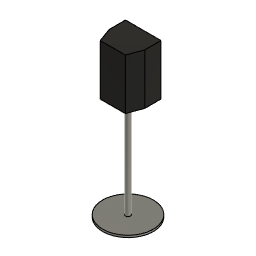
Speaker (Autodesk Fusion 360 design; units mm, degrees)
Autodesk Fusion 360 part; units mm, degrees
sketch "Schizzo1" plane through (0, 0, 0) normal (0, 0, 1) x (1, 0, 0)
  circle A0 centre (0, 0) radius 250
  dimension "d1" = 500
  constraint coincident A0.centre origin
  measures "d1" diameter of A0
extrude "Estrusione1" add sketch "Schizzo1" along normal blind 20
sketch "Schizzo2" plane through (0, 0, 20) normal (0, 0, 1) x (-1, 0, 0)
  circle A0 centre (0, 0) radius 250
  circle A1 centre (0, 0) radius 25
  dimension "d4" = 50
  constraint coincident A0.centre A1.centre
  measures "d4" diameter of A1
extrude "Estrusione2" add sketch "Schizzo2" along normal blind 1000 contours A1
sketch "Schizzo3" plane through (0, 0, 1020) normal (0, 0, 1) x (-1, 0, 0)
  circle A0 centre (0, 0) radius 25
  line L0 (-175, -150) -> (175, -150)
  line L1 (175, -150) -> (175, 150)
  line L2 (175, 150) -> (-175, 150)
  line L3 (-175, 150) -> (-175, -150)
  line L4 (-175, -150) -> (175, 150) construction
  line L5 (175, -150) -> (-175, 150) construction
  line L6 (-123.697, 150) -> (-175, 9.0461)
  line L7 (123.697, 150) -> (175, 9.0461)
  dimension "d7" = 350
  dimension "d8" = 300
  dimension "d11" = 150
  dimension "d12" = 20
  dimension "d13" = 20
  constraint horizontal L0
  constraint perpendicular L0 L1
  constraint parallel L0 L2
  constraint parallel L1 L3
  constraint coincident L4 A0.centre
  constraint coincident L5 A0.centre
  constraint coincident A0.centre origin
  constraint coincident L2 L6.start
  constraint coincident L3 L6.end
  constraint coincident L2 L7.start
  constraint coincident L1 L7.end
  constraint equal L6 L7
  measures "d7" distance of L1.end L2.end
  measures "d8" distance of L0.end L1.end
  measures "d11" distance of L6.start L6.end
  measures "d12" angle of L3 L6
  measures "d13" angle of L1 L7
extrude "Estrusione3" add sketch "Schizzo3" along normal blind 500 contours A0 | L0 L1 L2 L3 L6 L7
sketch "Schizzo4" plane through (0, 150, 0) normal (0, 1, 0) x (-1, 0, 0)
  line L0 (-175, 1020) -> (175, 1020)
  line L1 (175, 1020) -> (175, 1520)
  line L2 (175, 1520) -> (-175, 1520)
  line L3 (-175, 1520) -> (-175, 1020)
  line L4 (0, 1520) -> (0, 1020) construction
  circle A0 centre (0, 1420) radius 60
  circle A1 centre (0, 1180) radius 125
  dimension "d14" = 120
  dimension "d15" = 250
  dimension "d16" = 100
  dimension "d17" = 160
  constraint midpoint L2 L4.start
  constraint midpoint L0 L4.end
  constraint coincident L4 A0.centre
  constraint coincident L4 A1.centre
  measures "d14" diameter of A0
  measures "d15" diameter of A1
  measures "d16" distance of L2 A0.centre
  measures "d17" distance of L0 A1.centre
extrude "Estrusione4" cut sketch "Schizzo4" against normal blind 20 contours A0 | A1
component "Component" placed x (1, 0, 0) y (0, 1, 0) z (0, 0, 1) at (0, 0, 0)
